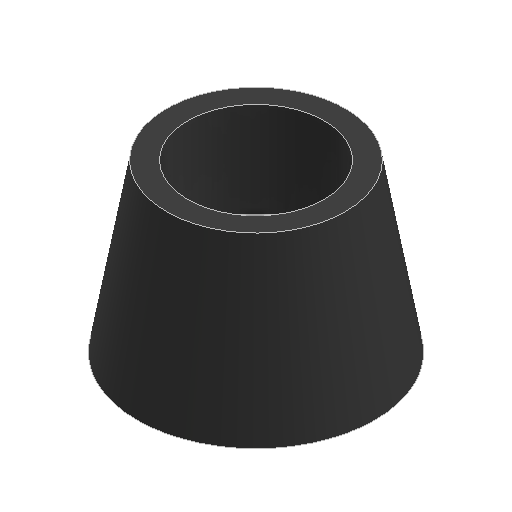
# Autodesk Inventor part: Foot
Saved by Autodesk Inventor 2026.2 (Build 302298000, 298)
## iProperties
Created: 2026-03-20
Part Number: Foot
Material: Rubber
Document SubType Name: Modeling
Designer: gaoet
Density: 0.93 g/cm^3
Appearance: Rubber - Black
Author: gaoet
Autodesk Inventor part; units mm, degrees
ref_plane "YZ Plane" through (0, 0, 0) normal (1, 0, 0) x (0, 1, 0)
ref_plane "XZ Plane" through (0, 0, 0) normal (0, 1, 0) x (-1, 0, 0)
ref_plane "XY Plane" through (0, 0, 0) normal (0, 0, 1) x (1, 0, 0)
sketch "Sketch1" plane through (0, 0, 0) normal (0, 0, 1) x (1, 0, 0)
  line L0 (0, 0) -> (0, 14.2576) construction
  line L1 (0, 0) -> (5, 0)
  line L2 (5, 0) -> (3.7657, 7)
  line L3 (3.7657, 7) -> (2.875, 7)
  line L4 (2.875, 7) -> (2.875, 3)
  line L5 (2.875, 3) -> (1.5, 3)
  line L6 (1.5, 3) -> (1.5, 0)
  point P0 (3.3204, 7)
  dimension "d0" = 1.5
  dimension "d1" = 2.875
  dimension "d2" = 7
  dimension "d3" = 4
  dimension "d4" = 80
  dimension "d5" = 5
  constraints: 14 end point, 2 horizontal, 2 vertical, 1 midpoint, 1 parallel, 1 perpendicular, 1 point on line
  measures "d0" distance between parallel lines of L0 L6
  measures "d1" distance between parallel lines of L0 L4
  measures "d2" distance from line of L1 point (3.32, 7)
  measures "d3" distance of L3.end L4.end
  measures "d4" angle of L1 L2
  measures "d5" distance of L0.start L1.end
revolve "Revolution1" add sketch "Sketch1" angle 360 about axis through (0, 0, 0) along (0, 1, 0)
body "Solid1"
